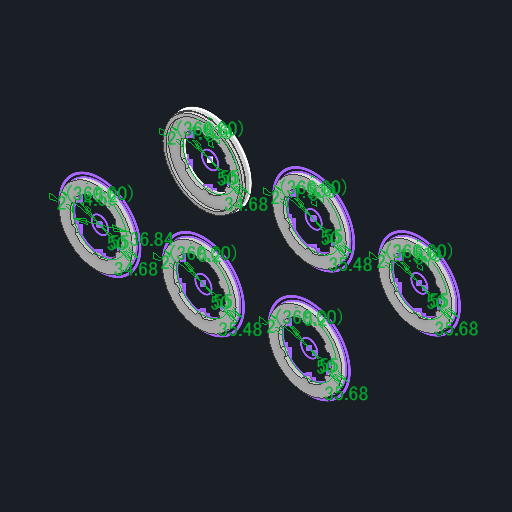
# Autodesk Inventor part: baicPart
Saved by Autodesk Inventor 2025.2 (Build 292293000, 293)
## iProperties
Company: FC-TORQUE
Created: 2025-03-14
Part Number: baicPart
Material: 一般
Document SubType Name: Modeling
Designer: Keito Tamura
Density: 1 g/cm^3
Appearance: 既定
Author: Keito Tamura
Autodesk Inventor part; units mm, degrees
ref_plane "YZ Plane" through (0, 0, 0) normal (1, 0, 0) x (0, 1, 0)
ref_plane "XZ Plane" through (0, 0, 0) normal (0, 1, 0) x (-1, 0, 0)
ref_plane "XY Plane" through (0, 0, 0) normal (0, 0, 1) x (1, 0, 0)
sketch "スケッチ1" plane through (0, 0, 0) normal (0, 0, 1) x (1, 0, 0)
  circle A0 centre (0, 0) radius 17.34
  circle A1 centre (0, 0) radius 5.5
  circle A2 centre (0, 0) radius 18.4198
  circle A3 centre (0, 18.4198) radius 2.8
  line L0 (-2.5, 17.1588) -> (2.5, 17.1588)
  line L1 (0, 15.6198) -> (0, 17.1588)
  circle A4 centre (-15.952, 9.2099) radius 2.8
  circle A5 centre (-15.952, -9.2099) radius 2.8
  circle A6 centre (0, -18.4198) radius 2.8
  circle A7 centre (15.952, -9.2099) radius 2.8
  circle A8 centre (15.952, 9.2099) radius 2.8
  circle A9 centre (0, 0) radius 0.9862
  circle A10 centre (0, 0) radius 25
  circle A11 centre (0, 0) radius 27
  circle A12 centre (0, 0) radius 27.5
  circle A13 centre (86.4856, 9.6457) radius 2.8
  circle A14 centre (53.8816, 9.6457) radius 2.8
  line L2 (70.1836, 16.2576) -> (70.1836, 17.7967)
  circle A15 centre (70.1836, 19.0576) radius 2.8
  line L3 (67.6836, 17.7967) -> (72.6836, 17.7967)
  circle A16 centre (70.1836, 0.2337) radius 18.8239
  circle A17 centre (70.1836, 0.2337) radius 17.74
  circle A18 centre (70.1836, 0.2337) radius 5.5
  circle A19 centre (86.4856, -9.1782) radius 2.8
  circle A20 centre (70.1836, -18.5902) radius 2.8
  circle A21 centre (53.8816, -9.1782) radius 2.8
  circle A22 centre (70.1836, 0.2337) radius 0.9862
  circle A23 centre (70.1836, 0.2337) radius 25
  circle A24 centre (70.1836, 0.2337) radius 27
  circle A25 centre (70.1836, 0.2337) radius 27.5
  circle A26 centre (158.3251, 7.9712) radius 2.8
  circle A27 centre (125.5462, 7.9712) radius 2.8
  line L4 (141.9357, 14.6336) -> (141.9357, 16.1727)
  circle A28 centre (141.9357, 17.4336) radius 2.8
  line L5 (139.4357, 16.1727) -> (144.4357, 16.1727)
  circle A29 centre (141.9357, -1.4913) radius 18.9249
  circle A30 centre (141.9357, -1.4913) radius 17.84
  circle A31 centre (141.9357, -1.4913) radius 5.5
  circle A32 centre (158.3251, -10.9537) radius 2.8
  circle A33 centre (141.9357, -20.4162) radius 2.8
  circle A34 centre (125.5462, -10.9538) radius 2.8
  circle A35 centre (141.9357, -1.4913) radius 0.9862
  circle A36 centre (141.9357, -1.4913) radius 25
  circle A37 centre (141.9357, -1.4913) radius 27
  circle A38 centre (141.9357, -1.4913) radius 27.5
  circle A39 centre (-58.7519, -66.2045) radius 2.6
  circle A40 centre (-90.6559, -66.2045) radius 2.6
  line L6 (-74.7039, -59.5946) -> (-74.7039, -58.2263)
  circle A41 centre (-74.7039, -56.9946) radius 2.6
  line L7 (-76.9937, -58.2263) -> (-72.4141, -58.2263)
  circle A42 centre (-74.7039, -75.4144) radius 18.4198
  circle A43 centre (-74.7039, -75.4144) radius 17.34
  circle A44 centre (-74.7039, -75.4144) radius 5.5
  circle A45 centre (-58.7519, -84.6243) radius 2.6
  circle A46 centre (-74.7039, -93.8342) radius 2.6
  circle A47 centre (-90.6559, -84.6243) radius 2.6
  circle A48 centre (-74.7039, -75.4144) radius 0.9862
  circle A49 centre (-74.7039, -75.4144) radius 25
  circle A50 centre (-74.7039, -75.4144) radius 27
  circle A51 centre (-74.7039, -75.4144) radius 27.5
  circle A52 centre (-4.5203, -75.1807) radius 5.5
  circle A53 centre (-4.5203, -75.1807) radius 17.74
  circle A54 centre (-4.5203, -75.1807) radius 18.2771
  circle A55 centre (-4.5203, -75.1807) radius 25
  circle A56 centre (-4.5203, -75.1807) radius 27.5
  circle A57 centre (-4.5203, -75.1807) radius 27
  circle A58 centre (11.3081, -66.0421) radius 2.6
  circle A59 centre (-4.5203, -75.1807) radius 0.9862
  circle A60 centre (11.3082, -84.3192) radius 2.6
  circle A61 centre (-4.5203, -93.4578) radius 2.6
  circle A62 centre (-20.3487, -66.0421) radius 2.6
  circle A63 centre (-20.3487, -84.3192) radius 2.6
  line L8 (-4.5203, -59.5036) -> (-4.5203, -57.6177)
  line L9 (-7.0203, -57.6177) -> (-2.0203, -57.6177)
  circle A64 centre (-4.5203, -56.9036) radius 2.6
  circle A65 centre (67.2318, -76.9057) radius 5.5
  circle A66 centre (67.2318, -76.9057) radius 17.84
  circle A67 centre (67.2318, -76.9057) radius 18.3781
  circle A68 centre (67.2318, -76.9057) radius 25
  circle A69 centre (67.2318, -76.9057) radius 27.5
  circle A70 centre (67.2318, -76.9057) radius 27
  circle A71 centre (83.1477, -67.7166) radius 2.6
  circle A72 centre (67.2318, -76.9057) radius 0.9862
  circle A73 centre (83.1477, -86.0948) radius 2.6
  circle A74 centre (67.2318, -95.2838) radius 2.6
  circle A75 centre (51.3159, -67.7166) radius 2.6
  circle A76 centre (51.3159, -86.0948) radius 2.6
  line L10 (67.2318, -61.1276) -> (67.2318, -59.2417)
  line L11 (64.7318, -59.2417) -> (69.7318, -59.2417)
  circle A77 centre (67.2318, -58.5276) radius 2.6
  point P0 (-0.3987, 0.1519)
  point P1 (-0.3987, 0.1519)
  point P2 (-0.3987, 0.1519)
  point P3 (-0.3987, 0.1519)
  point P4 (-0.3987, 0.1519)
  point P5 (-0.3987, 0.1519)
  point P6 (-0.3987, 0.1519)
  point P7 (-0.3987, 0.1519)
  point P8 (-0.3987, 0.1519)
  point P9 (-0.3987, 0.1519)
  point P10 (-0.3987, 0.1519)
  point P11 (-0.3987, 0.1519)
  point P12 (-0.3987, 0.1519)
  point P13 (-0.3987, 0.1519)
  point P14 (-0.3987, 0.1519)
  point P15 (-0.3987, 0.1519)
  point P16 (-0.3987, 0.1519)
  point P17 (-0.3987, 0.1519)
  point P18 (-0.3987, 0.1519)
  point P19 (-0.3987, 0.1519)
  point P20 (-0.3987, 0.1519)
  point P21 (-0.3987, 0.1519)
  point P22 (-0.3987, 0.1519)
  point P23 (-0.3987, 0.1519)
  point P24 (-0.3987, 0.1519)
  point P25 (-0.3987, 0.1519)
  point P26 (-0.3987, 0.1519)
  point P27 (-0.3987, 0.1519)
  point P28 (-0.3987, 0.1519)
  point P29 (-0.3987, 0.1519)
  point P30 (-0.3987, 0.1519)
  point P31 (-0.3987, 0.1519)
  point P32 (-0.3987, 0.1519)
  point P33 (-0.3987, 0.1519)
  point P34 (-0.3987, 0.1519)
  point P35 (-0.3987, 0.1519)
  point P36 (-0.3987, 0.1519)
  point P37 (-0.3987, 0.1519)
  point P38 (-0.3987, 0.1519)
  point P39 (-0.3987, 0.1519)
  point P40 (-0.3987, 0.1519)
  point P41 (-0.3987, 0.1519)
  point P42 (-0.3987, 0.1519)
  point P43 (-0.3987, 0.1519)
  point P44 (-0.3987, 0.1519)
  point P45 (-0.3987, 0.1519)
  point P46 (-0.3987, 0.1519)
  point P47 (-0.3987, 0.1519)
  point P48 (-0.3987, 0.1519)
  point P49 (-0.3987, 0.1519)
  point P50 (-0.3987, 0.1519)
  point P51 (-0.3987, 0.1519)
  point P52 (-0.3987, 0.1519)
  point P53 (-0.3987, 0.1519)
  point P54 (-0.3987, 0.1519)
  point P55 (-0.3987, 0.1519)
  point P56 (-0.3987, 0.1519)
  point P57 (-0.3987, 0.1519)
  point P58 (-0.3987, 0.1519)
  point P59 (-0.3987, 0.1519)
  point P60 (-0.3987, 0.1519)
  point P61 (-0.3987, 0.1519)
  point P62 (-0.3987, 0.1519)
  point P63 (-0.3987, 0.1519)
  point P64 (-0.3987, 0.1519)
  point P65 (-0.3987, 0.1519)
  point P66 (-0.3987, 0.1519)
  point P67 (-0.3987, 0.1519)
  point P68 (-0.3987, 0.1519)
  point P69 (-0.3987, 0.1519)
  point P70 (-0.3987, 0.1519)
  point P71 (-0.3987, 0.1519)
  point P72 (-0.3987, 0.1519)
  point P73 (-0.3987, 0.1519)
  point P74 (-0.3987, 0.1519)
  point P75 (-16.11, 6.4144)
  point P76 (-13.61, 10.7445)
  point P77 (-13.5271, 7.8099)
  point P78 (-13.61, -10.7445)
  point P79 (-16.11, -6.4144)
  point P80 (-13.5271, -7.8099)
  point P81 (2.5, -17.1588)
  point P82 (-2.5, -17.1588)
  point P83 (0, -15.6198)
  point P84 (16.11, -6.4144)
  point P85 (13.61, -10.7445)
  point P86 (13.5271, -7.8099)
  point P87 (13.61, 10.7445)
  point P88 (16.11, 6.4144)
  point P89 (13.5271, 7.8099)
  point P90 (16.11, 6.4144)
  point P91 (16.11, -6.4144)
  point P92 (13.61, -10.7445)
  point P93 (2.5, -17.1588)
  point P94 (-2.5, -17.1588)
  point P95 (-13.61, -10.7445)
  point P96 (-16.11, -6.4144)
  point P97 (-16.11, 6.4144)
  point P98 (-13.61, 10.7445)
  point P99 (13.61, 10.7445)
  point P100 (84.0607, 8.2457)
  point P101 (86.6436, 6.8501)
  point P102 (84.1436, 11.1803)
  point P103 (69.7849, 0.7897)
  point P104 (69.7849, 0.7897)
  point P105 (69.7849, 0.7897)
  point P106 (69.7849, 0.7897)
  point P107 (69.7849, 0.7897)
  point P108 (69.7849, 0.7897)
  point P109 (69.7849, 0.7897)
  point P110 (69.7849, 0.7897)
  point P111 (69.7849, 0.7897)
  point P112 (69.7849, 0.7897)
  point P113 (69.7849, 0.7897)
  point P114 (69.7849, 0.7897)
  point P115 (69.7849, 0.7897)
  point P116 (69.7849, 0.7897)
  point P117 (69.7849, 0.7897)
  point P118 (69.7849, 0.7897)
  point P119 (69.7849, 0.7897)
  point P120 (69.7849, 0.7897)
  point P121 (69.7849, 0.7897)
  point P122 (69.7849, 0.7897)
  point P123 (69.7849, 0.7897)
  point P124 (69.7849, 0.7897)
  point P125 (69.7849, 0.7897)
  point P126 (69.7849, 0.7897)
  point P127 (69.7849, 0.7897)
  point P128 (69.7849, 0.7897)
  point P129 (69.7849, 0.7897)
  point P130 (69.7849, 0.7897)
  point P131 (69.7849, 0.7897)
  point P132 (69.7849, 0.7897)
  point P133 (69.7849, 0.7897)
  point P134 (69.7849, 0.7897)
  point P135 (69.7849, 0.7897)
  point P136 (69.7849, 0.7897)
  point P137 (69.7849, 0.7897)
  point P138 (69.7849, 0.7897)
  point P139 (69.7849, 0.7897)
  point P140 (69.7849, 0.7897)
  point P141 (69.7849, 0.7897)
  point P142 (69.7849, 0.7897)
  point P143 (69.7849, 0.7897)
  point P144 (69.7849, 0.7897)
  point P145 (69.7849, 0.7897)
  point P146 (69.7849, 0.7897)
  point P147 (69.7849, 0.7897)
  point P148 (69.7849, 0.7897)
  point P149 (69.7849, 0.7897)
  point P150 (69.7849, 0.7897)
  point P151 (69.7849, 0.7897)
  point P152 (69.7849, 0.7897)
  point P153 (69.7849, 0.7897)
  point P154 (69.7849, 0.7897)
  point P155 (69.7849, 0.7897)
  point P156 (69.7849, 0.7897)
  point P157 (69.7849, 0.7897)
  point P158 (69.7849, 0.7897)
  point P159 (69.7849, 0.7897)
  point P160 (69.7849, 0.7897)
  point P161 (69.7849, 0.7897)
  point P162 (69.7849, 0.7897)
  point P163 (56.2236, 11.1803)
  point P164 (56.3065, 8.2457)
  point P165 (53.7236, 6.8501)
  point P166 (69.7849, 0.7897)
  point P167 (69.7849, 0.7897)
  point P168 (69.7849, 0.7897)
  point P169 (69.7849, 0.7897)
  point P170 (69.7849, 0.7897)
  point P171 (69.7849, 0.7897)
  point P172 (69.7849, 0.7897)
  point P173 (69.7849, 0.7897)
  point P174 (69.7849, 0.7897)
  point P175 (86.6436, -6.3827)
  point P176 (84.1436, -10.7128)
  point P177 (84.0607, -7.7782)
  point P178 (70.1836, -15.7902)
  point P179 (72.6836, -17.3292)
  point P180 (67.6836, -17.3292)
  point P181 (56.3065, -7.7782)
  point P182 (56.2236, -10.7128)
  point P183 (53.7236, -6.3827)
  point P184 (69.7849, 0.7897)
  point P185 (69.7849, 0.7897)
  point P186 (69.7849, 0.7897)
  point P187 (69.7849, 0.7897)
  point P188 (69.7849, 0.7897)
  point P189 (69.7849, 0.7897)
  point P190 (155.9003, 6.5712)
  point P191 (158.4831, 5.1756)
  point P192 (155.9831, 9.5058)
  point P193 (157.5628, -3.7915)
  point P194 (157.5628, -3.7915)
  point P195 (157.5628, -3.7915)
  point P196 (157.5628, -3.7915)
  point P197 (157.5628, -3.7915)
  point P198 (157.5628, -3.7915)
  point P199 (157.5628, -3.7915)
  dimension "d64" = 36.8396
  dimension "d2" = 34.68
  dimension "d3" = 5.6
  dimension "d4" = 5
  dimension "d5" = 1.5391
  dimension "d6" = 360
  dimension "d7" = 50
  dimension "d8" = 2
  dimension "d9" = 55
  dimension "d16" = 35.48
  dimension "d17" = 5.6
  dimension "d18" = 5
  dimension "d19" = 1.5391
  dimension "d20" = 360
  dimension "d21" = 50
  dimension "d22" = 2
  dimension "d23" = 55
  dimension "d26" = 35.68
  dimension "d27" = 5.6
  dimension "d28" = 5
  dimension "d29" = 1.5391
  dimension "d30" = 360
  dimension "d31" = 50
  dimension "d32" = 2
  dimension "d33" = 55
  dimension "d40" = 34.68
  dimension "d41" = 5.2
  dimension "d44" = 360
  dimension "d45" = 50
  dimension "d46" = 2
  dimension "d47" = 55
  dimension "d48" = 35.48
  dimension "d49" = 5.2
  dimension "d52" = 360
  dimension "d53" = 50
  dimension "d54" = 2
  dimension "d55" = 55
  dimension "d56" = 35.68
  dimension "d57" = 5.2
  dimension "d60" = 360
  dimension "d61" = 50
  dimension "d62" = 2
  dimension "d63" = 55
  dimension "d65" = 4.5796
  constraints: 120 point on circle, 72 centre point, 60 coincident, 24 end point, 12 concentric, 6 midpoint, 1 vertical alignment, 203 other
  measures "d2" diameter of A0
  measures "d3" diameter of A3
  measures "d4" distance of L0.start L0.end
  measures "d5" distance of L1.start L1.end
  measures "d7" diameter of A10
  measures "d8" radial gap between concentric circles of A10 A11
  measures "d9" diameter of A12
  measures "d16" diameter of A17
  measures "d17" diameter of A15
  measures "d18" distance of L3.start L3.end
  measures "d19" distance of L2.start L2.end
  measures "d21" diameter of A23
  measures "d22" radial gap between concentric circles of A23 A24
  measures "d23" diameter of A25
  measures "d26" diameter of A30
  measures "d27" diameter of A28
  measures "d28" distance of L5.start L5.end
  measures "d29" distance of L4.start L4.end
  measures "d31" diameter of A36
  measures "d32" radial gap between concentric circles of A36 A37
  measures "d33" diameter of A38
  measures "d40" diameter of A43
  measures "d41" diameter of A41
  measures "d45" diameter of A49
  measures "d46" radial gap between concentric circles of A49 A50
  measures "d47" diameter of A51
  measures "d48" diameter of A53
  measures "d49" diameter of A64
  measures "d53" diameter of A55
  measures "d54" radial gap between concentric circles of A55 A57
  measures "d55" diameter of A56
  measures "d56" diameter of A66
  measures "d57" diameter of A77
  measures "d61" diameter of A68
  measures "d62" radial gap between concentric circles of A68 A70
  measures "d63" diameter of A69
  measures "d65" distance of L7.start L7.end
extrude "押し出し1" add sketch "スケッチ1" along normal blind 3.2 contours L0 A0 | A3 A2 A8 A0 | A0 A3 A2 | A3 L1 L0 | L0 L1 A3 | A0 A4 A2 A3 | A8 A2 A0 | A0 A8 | A2 A3 | A4 A0 | A0 A4 A2 | A8 A2 A7 A0 | A8 A2 | A0 A5 A2 A4 | A2 A4 | A5 A0 | A0 A5 A2 | A7 A2 A0 | A0 A7 | A0 A6 A2 A5 | A2 A5 | A7 A2 A6 A0 | A7 A2 | A6 A0 | A0 A6 A2 | A2 A6 | A10 | A12
extrude "押し出し2" add sketch "スケッチ1" along normal blind 5 contours A11
extrude "押し出し3" add sketch "スケッチ1" along normal blind 2.9 contours A39 A42 | A42 A39 A43 | A39 A43 A41 A42 | A42 A45 A43 A39 | A43 A39 | A42 A41 | A41 A43 A42 | A41 L6 L7 | L7 A43 | A41 A43 A40 A42 | A45 A42 | A42 A45 A43 | A41 L7 L6 | A42 A40 | A40 A43 A42 | A43 A45 | A42 A46 A43 A45 | A40 A43 | A40 A43 A47 A42 | A46 A42 | A42 A46 A43 | A47 A43 A42 | A42 A47 | A43 A46 | A42 A47 A43 A46 | A47 A43 | A49 | L9 A53 | A64 A54 A58 A53 | A64 L8 L9 | A53 A64 A54 | L9 L8 A64 | A53 A62 A54 A64 | A58 A54 A53 | A53 A58 | A54 A64 | A62 A53 | A53 A62 A54 | A58 A54 A60 A53 | A58 A54 | A53 A63 A54 A62 | A54 A62 | A63 A53 | A53 A63 A54 | A60 A54 A53 | A53 A60 | A53 A61 A54 A63 | A54 A63 | A60 A54 A61 A53 | A60 A54 | A61 A53 | A53 A61 A54 | A54 A61 | A55
extrude "押し出し4" add sketch "スケッチ1" along normal blind 2.9 contours A13 A16 | A16 A13 A17 | A13 A17 A15 A16 | A16 A19 A17 A13 | A17 A13 | A16 A15 | A15 A17 A16 | A15 L2 L3 | L3 A17 | A15 A17 A14 A16 | A19 A16 | A16 A19 A17 | A15 L3 L2 | A16 A14 | A14 A17 A16 | A17 A19 | A16 A20 A17 A19 | A14 A17 | A14 A17 A21 A16 | A20 A16 | A16 A20 A17 | A21 A17 A16 | A16 A21 | A17 A20 | A16 A21 A17 A20 | A21 A17 | A23 | A26 A29 | A29 A26 A30 | A26 A30 A28 A29 | A29 A32 A30 A26 | A30 A26 | A29 A28 | A28 A30 A29 | A28 L4 L5 | L5 A30 | A28 A30 A27 A29 | A32 A29 | A29 A32 A30 | A28 L5 L4 | A29 A27 | A27 A30 A29 | A30 A32 | A29 A33 A30 A32 | A27 A30 | A27 A30 A34 A29 | A33 A29 | A29 A33 A30 | A34 A30 A29 | A29 A34 | A30 A33 | A29 A34 A30 A33 | A34 A30 | A36 | L11 A66 | A77 A67 A71 A66 | A77 L10 L11 | A66 A77 A67 | L11 L10 A77 | A66 A75 A67 A77 | A71 A67 A66 | A66 A71 | A67 A77 | A75 A66 | A66 A75 A67 | A71 A67 A73 A66 | A71 A67 | A66 A76 A67 A75 | A67 A75 | A76 A66 | A66 A76 A67 | A73 A67 A66 | A66 A73 | A66 A74 A67 A76 | A67 A76 | A73 A67 A74 A66 | A73 A67 | A74 A66 | A66 A74 A67 | A67 A74 | A68
